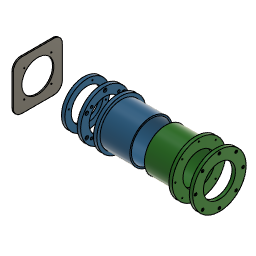
saturn-2-venting v14 (Autodesk Fusion 360 design; units mm, degrees)
Autodesk Fusion 360 part; units mm, degrees
sketch "mount-profile" plane through (0, 0, 0) normal (1, 0, 0) x (0, 1, 0)
  circle A0 centre (0, 0) radius 37.5
  circle A1 centre (-31.875, 31.875) radius 1.5
  line L0 (0, 0) -> (0, 37.5) construction
  line L1 (0, 0) -> (-37.5, 0) construction
  line L2 (-57.5, 57.5) -> (57.5, 57.5)
  line L3 (57.5, 57.5) -> (57.5, -57.5)
  line L4 (57.5, -57.5) -> (-57.5, -57.5)
  line L5 (-57.5, -57.5) -> (-57.5, 57.5)
  line L6 (0, 37.5) -> (0, 57.5) construction
  line L7 (-37.5, 0) -> (-57.5, 0) construction
  circle A2 centre (31.875, 31.875) radius 1.5
  circle A3 centre (-31.875, -31.875) radius 1.5
  circle A4 centre (31.875, -31.875) radius 1.5
  dimension "d1" = 75
  dimension "d2" = 3
  dimension "d7" = 20
  dimension "d8" = 20
  dimension "d9" = 20
  dimension "d10" = 20
  dimension "d13" = 30.375
  dimension "d14" = 30.375
  constraint coincident A0.centre L0.start
  constraint coincident A0 L0.end
  constraint vertical L0
  constraint coincident A0 L1.end
  constraint perpendicular L0 L1
  constraint horizontal L2
  constraint vertical L3
  constraint horizontal L4
  constraint vertical L5
  constraint midpoint L2 L6.end
  constraint midpoint L5 L7.end
  constraint symmetric A1 L6 A2
  constraint symmetric A1 L1 A3
  constraint symmetric L1 A2 A4
  measures "d1" diameter of A0
  measures "d2" diameter of A1
  measures "d7" distance of L0.end L2
  measures "d8" distance of A0 L3
  measures "d9" distance of A0 L4
  measures "d10" distance of L1.end L5
  measures "d13" distance of A1 L6
  measures "d14" distance of A1 L7
extrude "Extrude2" add sketch "mount-profile" along normal blind 3 makes body 1
sketch "saturn-outside" plane through (3, 0, 0) normal (1, 0, 0) x (0, 1, 0)
  circle A0 centre (-31.875, -31.875) radius 1.5
  circle A1 centre (-31.875, 31.875) radius 1.5
  circle A2 centre (31.875, 31.875) radius 1.5
  circle A3 centre (31.875, -31.875) radius 1.5
  circle A4 centre (0, 0) radius 37.5
  circle A5 centre (0, 0) radius 37.5
  circle A6 centre (0, 50) radius 4.05
  circle A7 centre (-43.3013, 25) radius 4.05
  circle A8 centre (-43.3013, -25) radius 4.05
  circle A9 centre (0, -50) radius 4.05
  circle A10 centre (43.3013, -25) radius 4.05
  circle A11 centre (43.3013, 25) radius 4.05
  circle A12 centre (0, 0) radius 62.5
  circle A13 centre (-31.875, 31.875) radius 1.5
  circle A14 centre (31.875, 31.875) radius 1.5
  circle A15 centre (31.875, -31.875) radius 1.5
  circle A16 centre (-31.875, -31.875) radius 1.5
  line L0 (0, 37.5) -> (0, 62.5) construction
  line L1 (0, 37.5) -> (50, 37.5) construction
  circle A17 centre (-31.875, 31.875) radius 2.875
  line L2 (0, 0) -> (37.5, 0) construction
  line L3 (0, 37.5) -> (0, 0) construction
  circle A18 centre (31.875, 31.875) radius 2.875
  circle A19 centre (-31.875, -31.875) radius 2.875
  circle A20 centre (31.875, -31.875) radius 2.875
  dimension "d27" = 8.1
  dimension "d30" = 360
  dimension "d33" = 125
  dimension "d39" = 5.75
  constraint coincident A5 L0.start
  constraint coincident A12 L0.end
  constraint vertical L0
  constraint midpoint A6.centre L0
  constraint coincident A12 L1.end
  constraint tangent A5 L1
  constraint perpendicular L0 L1
  constraint concentric A4 A12
  constraint concentric A13 A17
  constraint coincident A4.centre A5.centre
  constraint coincident A5 L2.end
  constraint horizontal L2
  constraint symmetric L0 A17 A18
  constraint symmetric A17 L2 A19
  constraint symmetric L2 A18 A20
  measures "d27" diameter of A6
  measures "d33" diameter of A12
  measures "d39" diameter of A17
extrude "Extrude5" add sketch "saturn-outside" along normal blind 8 separate body contours A6 | A7 | A8 | A9 | A10 | A11 | A12 | A17 | A18 | A19 | A20 makes body 2
extrude "Extrude6" cut sketch "saturn-outside" against normal blind 3.1 from surface at 8 contours A6 | A7 | A8 | A9 | A10 | A11 bodies 2
extrude "Extrude7" cut sketch "saturn-outside" against normal blind 3 from surface at 8 contours A17 | A18 | A19 | A20 bodies 2
fillet "Fillet2" radius 20 4 edges at (1.5, -57.5, 57.5) (1.5, -57.5, -57.5) (1.5, 57.5, -57.5) (1.5, 57.5, 57.5) on bodies 1
sketch "saturn-inside" plane through (11, 0, 0) normal (1, 0, 0) x (0, 1, 0)
  circle A0 centre (31.875, 31.875) radius 2.875
  circle A1 centre (31.875, -31.875) radius 2.875
  circle A2 centre (-31.875, 31.875) radius 2.875
  circle A3 centre (-31.875, -31.875) radius 2.875
  circle A4 centre (0, -50) radius 4.05
  circle A5 centre (0, 50) radius 4.05
  circle A6 centre (-43.3013, -25) radius 4.05
  circle A7 centre (43.3013, -25) radius 4.05
  circle A8 centre (43.3013, 25) radius 4.05
  circle A9 centre (-43.3013, 25) radius 4.05
  circle A10 centre (0, 0) radius 37.5
  circle A11 centre (0, 0) radius 62.5
  line L0 (-28.6996, 31.875) -> (-30.2873, 34.625)
  line L1 (-30.2873, 34.625) -> (-33.4627, 34.625)
  line L2 (-33.4627, 34.625) -> (-35.0504, 31.875)
  line L3 (-35.0504, 31.875) -> (-33.4627, 29.125)
  line L4 (-33.4627, 29.125) -> (-30.2873, 29.125)
  line L5 (-30.2873, 29.125) -> (-28.6996, 31.875)
  line L6 (0, 0) -> (0, 37.5) construction
  line L7 (0, 0) -> (-37.5, 0) construction
  line L8 (-31.875, 31.875) -> (-31.875, 34.75) construction
  line L9 (-35.0504, 31.875) -> (-31.875, 31.875) construction
  circle A12 centre (-31.875, 31.875) radius 1.5
  circle A13 centre (31.875, 31.875) radius 1.5
  line L10 (35.0504, 31.875) -> (33.4627, 29.125)
  line L11 (33.4627, 34.625) -> (35.0504, 31.875)
  line L12 (30.2873, 34.625) -> (33.4627, 34.625)
  line L13 (28.6996, 31.875) -> (30.2873, 34.625)
  line L14 (30.2873, 29.125) -> (28.6996, 31.875)
  line L15 (33.4627, 29.125) -> (30.2873, 29.125)
  line L16 (-33.4627, -29.125) -> (-30.2873, -29.125)
  line L17 (-35.0504, -31.875) -> (-33.4627, -29.125)
  line L18 (-33.4627, -34.625) -> (-35.0504, -31.875)
  line L19 (-30.2873, -34.625) -> (-33.4627, -34.625)
  line L20 (-28.6996, -31.875) -> (-30.2873, -34.625)
  line L21 (-30.2873, -29.125) -> (-28.6996, -31.875)
  circle A14 centre (-31.875, -31.875) radius 1.5
  circle A15 centre (31.875, -31.875) radius 1.5
  line L22 (30.2873, -29.125) -> (28.6996, -31.875)
  line L23 (28.6996, -31.875) -> (30.2873, -34.625)
  line L24 (30.2873, -34.625) -> (33.4627, -34.625)
  line L25 (33.4627, -34.625) -> (35.0504, -31.875)
  line L26 (35.0504, -31.875) -> (33.4627, -29.125)
  line L27 (33.4627, -29.125) -> (30.2873, -29.125)
  circle A16 centre (0, 0) radius 62.5
  circle A17 centre (0, 0) radius 37.5
  point P0 (-31.875, 31.875)
  dimension "d45" = 5.5
  constraint coincident P0 A2.centre
  constraint coincident A10.centre A11.centre
  constraint coincident A10 L6.end
  constraint vertical L6
  constraint coincident A10 L7.end
  constraint perpendicular L6 L7
  constraint coincident A2 L8.end
  constraint vertical L8
  constraint perpendicular L8 L9
  constraint symmetric L0.start L6 L13.start
  constraint symmetric L0.end L6 L12.start
  constraint symmetric L1.end L6 L11.start
  constraint symmetric L2.end L6 L10.start
  constraint symmetric L3.end L6 L10.end
  constraint symmetric L4.end L6 L14.start
  constraint symmetric L6 A12 A13
  constraint symmetric L0.start L7 L20.start
  constraint symmetric L0.end L7 L19.start
  constraint symmetric L1.end L7 L18.start
  constraint symmetric L2.end L7 L17.start
  constraint symmetric L3.end L7 L16.start
  constraint symmetric L4.end L7 L16.end
  constraint symmetric L7 A12 A14
  constraint symmetric L7 A13 A15
  constraint symmetric L7 L10.start L25.end
  constraint symmetric L7 L10.end L26.end
  constraint symmetric L7 L11.start L24.end
  constraint symmetric L7 L12.start L23.end
  constraint symmetric L7 L13.start L22.end
  constraint symmetric L7 L14.start L22.start
  measures "d45" distance of L0 L3
extrude "Extrude8" add sketch "saturn-inside" along normal blind 8 separate body contours A0 L10 L11 L12 L13 L14 L15 | A0 L10 L11 | A0 L11 | A0 L10 | A0 L11 L12 | A0 L10 L15 | A0 L12 | A0 L15 | A0 L12 L13 | A0 L14 L15 | A0 L13 | A0 L14 | A0 L13 L14 | A1 L22 L23 L24 L25 L26 L27 | A1 L25 L26 | A1 L26 | A1 L25 | A1 L26 L27 | A1 L24 L25 | A1 L27 | A1 L24 | A1 L22 L27 | A1 L23 L24 | A1 L22 | A1 L23 | A1 L22 L23 | A2 L0 L1 L2 L3 L4 L5 | A2 L0 L5 | A2 L0 | A2 L5 | A2 L0 L1 | A2 L4 L5 | A2 L1 | A2 L4 | A2 L1 L2 | A2 L3 L4 | A2 L2 | A2 L3 | A2 L2 L3 | A3 L16 L17 L18 L19 L20 L21 | A3 L20 L21 | A3 L21 | A3 L20 | A3 L16 L21 | A3 L19 L20 | A3 L16 | A3 L19 | A3 L16 L17 | A3 L18 L19 | A3 L17 | A3 L18 | A3 L17 L18 | A4 | A5 | A6 | A7 | A8 | A9 | A11 A16 makes body 3
extrude "Extrude9" cut sketch "saturn-inside" against normal blind 2.5 from surface at 8 contours A0 L10 L11 L12 L13 L14 L15 | A0 L10 L11 | A0 L11 L12 | A0 L10 L15 | A0 L12 L13 | A0 L14 L15 | A0 L13 L14 | A1 L22 L23 L24 L25 L26 L27 | A1 L25 L26 | A1 L26 L27 | A1 L24 L25 | A1 L22 L27 | A1 L23 L24 | A1 L22 L23 | A2 L0 L1 L2 L3 L4 L5 | A2 L0 L5 | A2 L0 L1 | A2 L4 L5 | A2 L1 L2 | A2 L3 L4 | A2 L2 L3 | A3 L16 L17 L18 L19 L20 L21 | A3 L20 L21 | A3 L16 L21 | A3 L19 L20 | A3 L16 L17 | A3 L18 L19 | A3 L17 L18 bodies 3
sketch "vent-to-saturn" plane through (11, 0, 0) normal (1, 0, 0) x (0, 1, 0)
  circle A0 centre (0, -50) radius 4.05
  circle A1 centre (0, 50) radius 4.05
  circle A2 centre (-43.3013, -25) radius 4.05
  circle A3 centre (43.3013, -25) radius 4.05
  circle A4 centre (43.3013, 25) radius 4.05
  circle A5 centre (-43.3013, 25) radius 4.05
  circle A6 centre (0, 0) radius 37.5
  circle A7 centre (0, 0) radius 62.5
  circle A8 centre (0, 0) radius 62.5
  circle A9 centre (0, 0) radius 37.5
  circle A10 centre (-43.3013, 25) radius 4.05
  circle A11 centre (0, 50) radius 4.05
  circle A12 centre (43.3013, 25) radius 4.05
  circle A13 centre (43.3013, -25) radius 4.05
  circle A14 centre (0, -50) radius 4.05
  circle A15 centre (-43.3013, -25) radius 4.05
  circle A16 centre (0, 0) radius 50
  circle A17 centre (0, 0) radius 46.5
  dimension "d55" = 100
  dimension "d56" = -3.5
  constraint concentric A9 A16
  measures "d55" diameter of A16
extrude "Extrude10" add sketch "vent-to-saturn" along normal blind 8 separate body contours A0 A14 A16 | A0 A14 A16 A17 | A0 A3 A13 A14 A16 A17 | A0 A2 A14 A15 A16 A17 | A0 A14 A17 | A0 A1 A2 A3 A4 A5 A10 A11 A12 A13 A14 A15 A17 | A3 A13 A16 | A3 A13 A16 A17 | A2 A15 A16 A17 | A2 A15 A16 | A3 A13 A17 | A3 A4 A12 A13 A16 A17 | A2 A15 A17 | A2 A5 A10 A15 A16 A17 | A5 A10 A16 A17 | A5 A10 A16 | A4 A12 A16 | A4 A12 A16 A17 | A5 A10 A17 | A1 A5 A10 A11 A16 A17 | A4 A12 A17 | A1 A4 A11 A12 A16 A17 | A1 A11 A16 A17 | A1 A11 A16 | A1 A11 A17 | A7 A8 makes body 4
extrude "Extrude11" cut sketch "vent-to-saturn" along normal blind 3.1 contours A0 A14 A16 | A0 A14 A16 A17 | A0 A14 A17 | A3 A13 A16 | A3 A13 A16 A17 | A2 A15 A16 A17 | A2 A15 A16 | A3 A13 A17 | A2 A15 A17 | A5 A10 A16 A17 | A5 A10 A16 | A4 A12 A16 | A4 A12 A16 A17 | A5 A10 A17 | A4 A12 A17 | A1 A11 A16 A17 | A1 A11 A16 | A1 A11 A17 bodies 4
extrude "Extrude12" add sketch "vent-to-saturn" along normal blind 70 from surface at 8 contours A0 A14 A16 A17 | A0 A3 A13 A14 A16 A17 | A0 A2 A14 A15 A16 A17 | A3 A13 A16 A17 | A2 A15 A16 A17 | A3 A4 A12 A13 A16 A17 | A2 A5 A10 A15 A16 A17 | A5 A10 A16 A17 | A4 A12 A16 A17 | A1 A5 A10 A11 A16 A17 | A1 A4 A11 A12 A16 A17 | A1 A11 A16 A17 bodies 4
move_body "Move2" bodies 4 to x (1, 0, 0) y (0, 1, 0) z (0, 0, 1) at (50, 0, 0)
move_body "Move3" bodies 3 to x (1, 0, 0) y (0, 1, 0) z (0, 0, 1) at (-50, 0, 0)
move_body "Move5" bodies 4 to x (1, 0, 0) y (0, 1, 0) z (0, 0, 1) at (-20, 0, 0)
move_body "Move6" bodies 3 to x (-1, 0, 0) y (0, -0.868456, -0.495766) z (0, -0.495766, 0.868456) at (-70, 0, 0)
sketch "vent-to-window" plane through (41, 0, 0) normal (-1, 0, 0) x (0, -1, 0)
  circle A0 centre (0, 0) radius 62.5
  circle A1 centre (0, 0) radius 62.5
  circle A2 centre (0, 0) radius 46.5
  circle A3 centre (0, 0) radius 50
  line L0 (0, 0) -> (0, 46.5) construction
  line L1 (0, 0) -> (46.5, 0) construction
  circle A4 centre (0, 0) radius 37.5
  line L2 (0, 46.5) -> (0, 62.5) construction
  circle A5 centre (0, 55.625) radius 1.5
  circle A6 centre (0, 55.625) radius 2.875
  circle A7 centre (-39.3328, 39.3328) radius 2.875
  circle A8 centre (-39.3328, 39.3328) radius 1.5
  circle A9 centre (-55.625, 0) radius 2.875
  circle A10 centre (-55.625, 0) radius 1.5
  circle A11 centre (-39.3328, -39.3328) radius 2.875
  circle A12 centre (-39.3328, -39.3328) radius 1.5
  circle A13 centre (0, -55.625) radius 2.875
  circle A14 centre (0, -55.625) radius 1.5
  circle A15 centre (39.3328, -39.3328) radius 2.875
  circle A16 centre (39.3328, -39.3328) radius 1.5
  circle A17 centre (55.625, 0) radius 2.875
  circle A18 centre (55.625, 0) radius 1.5
  circle A19 centre (39.3328, 39.3328) radius 2.875
  circle A20 centre (39.3328, 39.3328) radius 1.5
  line L3 (2.75, 54.0373) -> (2.75, 57.2127)
  line L4 (2.75, 57.2127) -> (0, 58.8004)
  line L5 (0, 58.8004) -> (-2.75, 57.2127)
  line L6 (-2.75, 57.2127) -> (-2.75, 54.0373)
  line L7 (-2.75, 54.0373) -> (0, 52.4496)
  line L8 (0, 52.4496) -> (2.75, 54.0373)
  line L9 (-38.511, 42.4) -> (-41.5782, 41.5782)
  line L10 (-41.5782, 41.5782) -> (-42.4, 38.511)
  line L11 (-42.4, 38.511) -> (-40.1547, 36.2656)
  line L12 (-40.1547, 36.2656) -> (-37.0874, 37.0874)
  line L13 (-37.0874, 37.0874) -> (-36.2656, 40.1547)
  line L14 (-36.2656, 40.1547) -> (-38.511, 42.4)
  line L15 (-57.2127, 2.75) -> (-58.8004, 0)
  line L16 (-58.8004, 0) -> (-57.2127, -2.75)
  line L17 (-57.2127, -2.75) -> (-54.0373, -2.75)
  line L18 (-54.0373, -2.75) -> (-52.4496, 0)
  line L19 (-52.4496, 0) -> (-54.0373, 2.75)
  line L20 (-54.0373, 2.75) -> (-57.2127, 2.75)
  line L21 (-42.4, -38.511) -> (-41.5782, -41.5782)
  line L22 (-41.5782, -41.5782) -> (-38.511, -42.4)
  line L23 (-38.511, -42.4) -> (-36.2656, -40.1547)
  line L24 (-36.2656, -40.1547) -> (-37.0874, -37.0874)
  line L25 (-37.0874, -37.0874) -> (-40.1547, -36.2656)
  line L26 (-40.1547, -36.2656) -> (-42.4, -38.511)
  line L27 (-2.75, -57.2127) -> (0, -58.8004)
  line L28 (0, -58.8004) -> (2.75, -57.2127)
  line L29 (2.75, -57.2127) -> (2.75, -54.0373)
  line L30 (2.75, -54.0373) -> (0, -52.4496)
  line L31 (0, -52.4496) -> (-2.75, -54.0373)
  line L32 (-2.75, -54.0373) -> (-2.75, -57.2127)
  line L33 (38.511, -42.4) -> (41.5782, -41.5782)
  line L34 (41.5782, -41.5782) -> (42.4, -38.511)
  line L35 (42.4, -38.511) -> (40.1547, -36.2656)
  line L36 (40.1547, -36.2656) -> (37.0874, -37.0874)
  line L37 (37.0874, -37.0874) -> (36.2656, -40.1547)
  line L38 (36.2656, -40.1547) -> (38.511, -42.4)
  line L39 (57.2127, -2.75) -> (58.8004, 0)
  line L40 (58.8004, 0) -> (57.2127, 2.75)
  line L41 (57.2127, 2.75) -> (54.0373, 2.75)
  line L42 (54.0373, 2.75) -> (52.4496, 0)
  line L43 (52.4496, 0) -> (54.0373, -2.75)
  line L44 (54.0373, -2.75) -> (57.2127, -2.75)
  line L45 (42.4, 38.511) -> (41.5782, 41.5782)
  line L46 (41.5782, 41.5782) -> (38.511, 42.4)
  line L47 (38.511, 42.4) -> (36.2656, 40.1547)
  line L48 (36.2656, 40.1547) -> (37.0874, 37.0874)
  line L49 (37.0874, 37.0874) -> (40.1547, 36.2656)
  line L50 (40.1547, 36.2656) -> (42.4, 38.511)
  circle A21 centre (0, 0) radius 41
  point P0 (0, 55.625)
  dimension "d76" = 3
  dimension "d77" = 5.75
  dimension "d78" = 4
  dimension "d80" = 360
  dimension "d90" = 5.5
  dimension "d92" = 360
  dimension "d99" = 3.5
  constraint coincident A0.centre A1.centre
  constraint coincident A2 L0.end
  constraint vertical L0
  constraint coincident A2 L1.end
  constraint perpendicular L0 L1
  constraint coincident A1 L2.end
  constraint parallel L0 L2
  constraint coincident L2 P0
  constraint concentric A5 A6
  constraint coincident P0 A5.centre
  constraint coincident L2 L4.end
  measures "d76" diameter of A5
  measures "d77" diameter of A6
  measures "d90" distance of L5 L8
extrude "Extrude16" add sketch "vent-to-window" along normal blind 8 separate body contours A0 A1 | A2 | A3 | A5 | A6 L3 | A6 L3 L4 L5 L6 L7 L8 | A6 L3 L4 | A6 L3 L8 | A6 L4 | A6 L8 | A6 L4 L5 | A6 L7 L8 | A6 L5 | A6 L7 | A6 L5 L6 | A6 L6 L7 | A6 L6 | A7 L13 | A7 L9 L10 L11 L12 L13 L14 | A7 L13 L14 | A7 L12 L13 | A7 L14 | A7 L12 | A7 L9 L14 | A7 L11 L12 | A7 L9 | A7 L11 | A7 L9 L10 | A7 L10 L11 | A7 L10 | A8 | A9 L15 L16 L17 L18 L19 L20 | A9 L18 L19 | A9 L19 | A9 L18 | A9 L19 L20 | A9 L17 L18 | A9 L20 | A9 L17 | A9 L15 L20 | A9 L16 L17 | A9 L15 | A9 L16 | A9 L15 L16 | A10 | A11 L24 | A11 L21 L22 L23 L24 L25 L26 | A11 L24 L25 | A11 L23 L24 | A11 L25 | A11 L23 | A11 L25 L26 | A11 L22 L23 | A11 L26 | A11 L22 | A11 L21 L26 | A11 L21 L22 | A11 L21 | A12 | A13 L29 | A13 L27 L28 L29 L30 L31 L32 | A13 L29 L30 | A13 L28 L29 | A13 L30 | A13 L28 | A13 L30 L31 | A13 L27 L28 | A13 L31 | A13 L27 | A13 L31 L32 | A13 L27 L32 | A13 L32 | A14 | A15 L34 | A15 L33 L34 L35 L36 L37 L38 | A15 L34 L35 | A15 L33 L34 | A15 L35 | A15 L33 | A15 L35 L36 | A15 L33 L38 | A15 L36 | A15 L38 | A15 L36 L37 | A15 L37 L38 | A15 L37 | A16 | A17 L39 L40 L41 L42 L43 L44 | A17 L39 L40 | A17 L40 | A17 L39 | A17 L40 L41 | A17 L39 L44 | A17 L41 | A17 L44 | A17 L41 L42 | A17 L43 L44 | A17 L42 | A17 L43 | A17 L42 L43 | A18 | A19 L45 | A19 L45 L46 L47 L48 L49 L50 | A19 L45 L46 | A19 L45 L50 | A19 L46 | A19 L50 | A19 L46 L47 | A19 L49 L50 | A19 L47 | A19 L49 | A19 L47 L48 | A19 L48 L49 | A19 L48 | A20 | A21 makes body 5
move_body "Move7" bodies 5 to x (1, 0, 0) y (0, 1, 0) z (0, 0, 1) at (330, 0, 0)
extrude "Extrude17" add 1 faces at (119, 48.4741, 4.7942) along direction (-1, 0, 0) blind 70 from surface at -244 on bodies 4 bodies 4 5
extrude "Extrude18" cut sketch "vent-to-window" against normal up to surface (8 mm away) from surface at -322 contours A5 | A8 | A10 | A12 | A14 | A16 | A18 | A20 bodies 5
extrude "Extrude19" add sketch "vent-to-window" against normal blind 8 from surface at -330 separate body contours A0 A1 | A6 L3 | A6 L3 L4 L5 L6 L7 L8 | A6 L3 L4 | A6 L3 L8 | A6 L4 | A6 L8 | A6 L4 L5 | A6 L7 L8 | A6 L5 | A6 L7 | A6 L5 L6 | A6 L6 L7 | A6 L6 | A7 L13 | A7 L9 L10 L11 L12 L13 L14 | A7 L13 L14 | A7 L12 L13 | A7 L14 | A7 L12 | A7 L9 L14 | A7 L11 L12 | A7 L9 | A7 L11 | A7 L9 L10 | A7 L10 L11 | A7 L10 | A9 L15 L16 L17 L18 L19 L20 | A9 L18 L19 | A9 L19 | A9 L18 | A9 L19 L20 | A9 L17 L18 | A9 L20 | A9 L17 | A9 L15 L20 | A9 L16 L17 | A9 L15 | A9 L16 | A9 L15 L16 | A11 L24 | A11 L21 L22 L23 L24 L25 L26 | A11 L24 L25 | A11 L23 L24 | A11 L25 | A11 L23 | A11 L25 L26 | A11 L22 L23 | A11 L26 | A11 L22 | A11 L21 L26 | A11 L21 L22 | A11 L21 | A13 L29 | A13 L27 L28 L29 L30 L31 L32 | A13 L29 L30 | A13 L28 L29 | A13 L30 | A13 L28 | A13 L30 L31 | A13 L27 L28 | A13 L31 | A13 L27 | A13 L31 L32 | A13 L27 L32 | A13 L32 | A15 L34 | A15 L33 L34 L35 L36 L37 L38 | A15 L34 L35 | A15 L33 L34 | A15 L35 | A15 L33 | A15 L35 L36 | A15 L33 L38 | A15 L36 | A15 L38 | A15 L36 L37 | A15 L37 L38 | A15 L37 | A17 L39 L40 L41 L42 L43 L44 | A17 L39 L40 | A17 L40 | A17 L39 | A17 L40 L41 | A17 L39 L44 | A17 L41 | A17 L44 | A17 L41 L42 | A17 L43 L44 | A17 L42 | A17 L43 | A17 L42 L43 | A19 L45 | A19 L45 L46 L47 L48 L49 L50 | A19 L45 L46 | A19 L45 L50 | A19 L46 | A19 L50 | A19 L46 L47 | A19 L49 L50 | A19 L47 | A19 L49 | A19 L47 L48 | A19 L48 L49 | A19 L48 makes body 6
move_body "Move8" bodies 6 to x (1, 0, 0) y (0, 1, 0) z (0, 0, 1) at (40, 0, 0)
extrude "Extrude20" cut sketch "vent-to-window" against normal blind 2.25 from surface at -322 contours A6 L3 | A6 L3 L4 L5 L6 L7 L8 | A6 L4 | A6 L8 | A6 L5 | A6 L7 | A6 L6 | A7 L9 L10 L11 L12 L13 L14 | A7 L14 | A7 L12 | A7 L9 | A7 L11 | A7 L10 | A9 L15 L16 L17 L18 L19 L20 | A9 L19 | A9 L18 | A9 L20 | A9 L17 | A9 L15 | A9 L16 | A11 L21 L22 L23 L24 L25 L26 | A11 L23 | A11 L25 | A11 L22 | A11 L26 | A11 L21 | A13 L29 | A13 L27 L28 L29 L30 L31 L32 | A13 L30 | A13 L28 | A13 L31 | A13 L27 | A13 L32 | A15 L33 L34 L35 L36 L37 L38 | A15 L35 | A15 L33 | A15 L36 | A15 L38 | A15 L37 | A17 L39 L40 L41 L42 L43 L44 | A17 L40 | A17 L39 | A17 L41 | A17 L44 | A17 L42 | A17 L43 | A19 L45 L46 L47 L48 L49 L50 | A19 L50 | A19 L46 | A19 L49 | A19 L47 | A19 L48 bodies 5
extrude "Extrude21" cut sketch "vent-to-window" along normal blind 2.5 from surface at -378 contours A6 L3 L4 L5 L6 L7 L8 | A6 L3 L4 | A6 L3 L8 | A6 L4 L5 | A6 L7 L8 | A6 L5 L6 | A6 L6 L7 | A7 L9 L10 L11 L12 L13 L14 | A7 L13 L14 | A7 L12 L13 | A7 L9 L14 | A7 L11 L12 | A7 L9 L10 | A7 L10 L11 | A9 L15 L16 L17 L18 L19 L20 | A9 L18 L19 | A9 L19 L20 | A9 L17 L18 | A9 L15 L20 | A9 L16 L17 | A9 L15 L16 | A11 L21 L22 L23 L24 L25 L26 | A11 L24 L25 | A11 L23 L24 | A11 L25 L26 | A11 L22 L23 | A11 L21 L26 | A11 L21 L22 | A13 L27 L28 L29 L30 L31 L32 | A13 L29 L30 | A13 L28 L29 | A13 L30 L31 | A13 L27 L28 | A13 L31 L32 | A13 L27 L32 | A15 L33 L34 L35 L36 L37 L38 | A15 L34 L35 | A15 L33 L34 | A15 L35 L36 | A15 L33 L38 | A15 L36 L37 | A15 L37 L38 | A17 L39 L40 L41 L42 L43 L44 | A17 L39 L40 | A17 L40 L41 | A17 L39 L44 | A17 L41 L42 | A17 L43 L44 | A17 L42 L43 | A19 L45 L46 L47 L48 L49 L50 | A19 L45 L46 | A19 L45 L50 | A19 L46 L47 | A19 L49 L50 | A19 L47 L48 | A19 L48 L49 bodies 6
move_body "Move9" bodies 5 6 to x (1, 0, 0) y (0, 1, 0) z (0, 0, 1) at (-140, 0, 0)
extrude "Extrude22" add sketch "vent-to-window" against normal up to surface (8 mm away) from surface at -230 contours A2 | A3 | A21 bodies 6
sketch "Sketch11" plane through (41, 0, 0) normal (-1, 0, 0) x (0, -1, 0)
  circle A0 centre (0, -50) radius 4.05
  circle A1 centre (0, 50) radius 4.05
  circle A2 centre (43.3013, -25) radius 4.05
  circle A3 centre (-43.3013, -25) radius 4.05
  circle A4 centre (-43.3013, 25) radius 4.05
  circle A5 centre (43.3013, 25) radius 4.05
  circle A6 centre (0, 0) radius 37.5
  circle A7 centre (0, 0) radius 62.5
  circle A8 centre (0, 0) radius 62.5
  circle A9 centre (0, 0) radius 37.5
  circle A10 centre (0, 50) radius 4.05
  circle A11 centre (43.3013, 25) radius 4.05
  circle A12 centre (43.3013, -25) radius 4.05
  circle A13 centre (-43.3013, 25) radius 4.05
  circle A14 centre (-43.3013, -25) radius 4.05
  circle A15 centre (0, -50) radius 4.05
  circle A16 centre (0, 50) radius 4.375
  circle A17 centre (-43.3013, 25) radius 4.375
  circle A18 centre (-43.3013, -25) radius 4.375
  circle A19 centre (0, -50) radius 4.375
  circle A20 centre (43.3013, -25) radius 4.375
  circle A21 centre (43.3013, 25) radius 4.375
  point P0 (-39.2513, 25)
  dimension "d105" = 8.75
  dimension "d107" = 360
  constraint concentric A10 A16
  measures "d105" diameter of A16
extrude "Extrude24" cut sketch "Sketch11" against normal up to surface (3.1 mm away) contours A16 | A17 | A18 | A19 | A20 | A21 bodies 4
sketch "Sketch12" plane through (119, 0, 0) normal (1, 0, 0) x (0, 1, 0)
  circle A0 centre (0, 0) radius 46.5
  circle A1 centre (0, 0) radius 50
  circle A2 centre (0, 0) radius 50
  circle A3 centre (0, 0) radius 51.75
  dimension "d110" = 1.75
move_face "OffsetFaces1" offset -10 1 faces at (-36.3333, 50.9236, 36.2358) on bodies 3
move_face "OffsetFaces2" offset -5 2 faces at (8.3333, -62.4223, 3.1154) (43.6667, -62.4223, 3.1154) on bodies 2 4
move_body "Move10" bodies 1 to x (1, 0, 0) y (0, 1, 0) z (0, 0, 1) at (-150, 0, 0)
equation "d13 = ( 60.75 / 2 ) * 1 mm"
equation "d14 = ( 60.75 / 2 ) * 1 mm"
named bodies: "mount-test", "saturn-outside", "saturn-inside", "vent-to-saturn", "vent-inside", "vent-outside"
